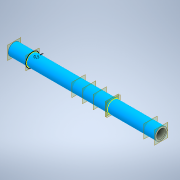
# Autodesk Inventor part: eje_solo
Saved by Autodesk Inventor 2021 (Build 250183000, 183)
## iProperties
Created: 2021-12-11
Part Number: eje_solo
Material: Generic
Document SubType Name: Modeling
Designer: Juan M. Casillas
Density: 1 g/cm^3
Appearance: Default
Author: Juan M. Casillas
Autodesk Inventor part; units mm, degrees
ref_plane "YZ Plane" through (0, 0, 0) normal (1, 0, 0) x (0, 1, 0)
ref_plane "XZ Plane" through (0, 0, 0) normal (0, 1, 0) x (-1, 0, 0)
ref_plane "XY Plane" through (0, 0, 0) normal (0, 0, 1) x (1, 0, 0)
sketch "Sketch1" plane through (0, 0, 0) normal (1, 0, 0) x (0, 1, 0)
  circle A0 centre (0, 0) radius 4
  dimension "d0" = 8
  constraints: 1 centre point, 1 coincident
  measures "d0" diameter of A0
extrude "Extrusion1" add sketch "Sketch1" along normal blind 97
sketch "Sketch2" plane through (97, 0, 0) normal (1, 0, 0) x (0, 0, -1)
  circle A0 centre (0, 0) radius 4 projected
  circle A1 centre (0, 0) radius 3
  dimension "d3" = 1
  constraints: 1 centre point
  measures "d3" radial gap between concentric circles of A0 A1
extrude "Extrusion2" cut sketch "Sketch2" against normal through all contours A1
ref_plane "Work Plane4" through (49.5, 0, 0) normal (-1, 0, 0) x (0, 0, 1)
ref_plane "Work Plane3" through (42.5, 0, 0) normal (-1, 0, 0) x (0, 0, 1)
ref_plane "Work Plane6" through (64.5, 0, 0) normal (-1, 0, 0) x (0, 0, 1)
ref_plane "Work Plane5" through (56.5, 0, 0) normal (-1, 0, 0) x (0, 0, 1)
ref_plane "Work Plane7" through (64.5, 0, 0) normal (-1, 0, 0) x (0, 0, 1)
sketch "Sketch3" plane through (12, 0, 0) normal (-1, 0, 0) x (0, 0, 1)
  circle A0 centre (0, 0) radius 4 projected
  circle A1 centre (0, 0) radius 4 projected
  circle A2 centre (0, 0) radius 4.5
  dimension "d13" = 0.5
  constraints: 1 centre point
  measures "d13" radial gap between concentric circles of A0 A2
ref_plane "Work Plane9" through (97, 0, 0) normal (-1, 0, 0) x (0, 0, 1)
ref_plane "Work Plane8" through (90, 0, 0) normal (-1, 0, 0) x (0, 0, 1)
ref_plane "Work Plane11" through (65.5, 0, 0) normal (-1, 0, 0) x (0, 0, 1)
sketch "Sketch5" plane through (65.5, 0, 0) normal (-1, 0, 0) x (0, 0, 1)
  circle A0 centre (0, 0) radius 4 projected
  circle A1 centre (0, 0) radius 4 projected
ref_plane "Work Plane1" through (0, 0, 0) normal (-1, 0, 0) x (0, 0, 1)
ref_plane "Work Plane2" through (12, 0, 0) normal (-1, 0, 0) x (0, 0, 1)
body "Solid1"
